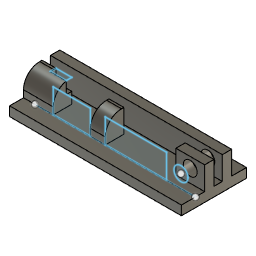
LM2596 Card Mount v10 (Autodesk Fusion 360 design; units mm, degrees)
Autodesk Fusion 360 part; units mm, degrees
note: some values were not read from the file. Chosen so that the rebuilt part matches the saved one: a direction; which face or edge a step refers to.
imported_body "Base Feature1'" makes body 1
sketch "Sketch1" plane through (0, 0, 0) normal (1, 0, 0) x (0, 1, 0)
  line L0 (7.8, 0) -> (0, 0)
  line L1 (0, 0) -> (0, 3.5)
  line L2 (3.5, 7) -> (7.8, 7)
  line L3 (7.8, 7) -> (7.8, 0)
  arc A0 (3.5, 7) -> (0, 3.5) centre (3.5, 3.5) ccw
  line L4 (4, 7) -> (4, 2)
  line L5 (4, 2) -> (5.8, 2)
  line L6 (5.8, 2) -> (5.8, 7)
  line L7 (4, 2) -> (0, 2) construction
  line L8 (4, 7) -> (2, 7)
  line L9 (2, 7) -> (2, 2)
  line L10 (2, 2) -> (4, 2)
  line L11 (4, 2) -> (4, 7)
  dimension "d9" = 7
  dimension "d11" = 3.5
  dimension "d12" = 4
  dimension "d13" = 1.8
  dimension "d27" = 2
  dimension "d37" = 2
  dimension "d50" = 2
  constraint horizontal L0
  constraint vertical L1
  constraint horizontal L2
  constraint vertical L3
  constraint tangent L1 A0
  constraint tangent L2 A0
  constraint coincident L2 L4.start
  constraint perpendicular L2 L4
  constraint perpendicular L4 L5
  constraint coincident L2 L6.end
  constraint perpendicular L2 L6
  constraint coincident L0.end L1.start
  constraint coincident L1 L7.end
  constraint collinear L5 L7
  constraint horizontal L8
  constraint vertical L9
  constraint horizontal L10
  constraint vertical L11
  measures "d9" distance of L0.start L2.end
  measures "d11" radius of A0
  measures "d12" distance of L1.end L4
  measures "d13" distance of L4 L6
  measures "d27" distance of L0 L5
  measures "d37" distance of L3 L6
  measures "d50" distance of L4.start L8.end
extrude "Extrude1" add sketch "Sketch1" along normal blind 37 separate body contours L0 L1 L2 L3 A0 L5 L6 L9 L10 | L2 A0 L4 L8 L9 L10 L11 sketch seen with x (1, 0, 0) y (0, 0, -1) z (0, 1, 0) at (0, -1.7661, 8.5008) makes body 2
sketch "Sketch2" plane through (0, 0, 0) normal (0, 1, 0) x (1, 0, 0)
  line L0 (6.4, -7.2451) -> (14.4, -7.2451)
  line L1 (14.4, -7.2451) -> (14.4, -2)
  line L2 (14.4, -2) -> (6.4, -2)
  line L3 (6.4, -2) -> (6.4, -7.2451)
  line L4 (17.6, -7.2451) -> (30.8, -7.2451)
  line L5 (30.8, -7.2451) -> (30.8, -2)
  line L6 (30.8, -2) -> (17.6, -2)
  line L7 (17.6, -2) -> (17.6, -7.2451)
  circle A0 centre (33.9, -4.8) radius 1.5
  line L8 (2.4997, -2) -> (37, -2)
  dimension "d16" = 3
  dimension "d17" = 2.8
  dimension "d24" = 2
  dimension "d34" = 13.2
  dimension "d35" = 3.2
  dimension "d36" = 8
  dimension "d53" = 6.2
  constraint perpendicular L3 L8
  constraint collinear L0 L4
  constraint collinear L2 L8
  constraint collinear L6 L8
  measures "d16" diameter of A0
  measures "d17" distance of L6 A0.centre
  measures "d24" distance of origin L8
  measures "d34" distance of L5 L7
  measures "d35" distance of L1 L7
  measures "d36" distance of L1 L3
  measures "d53" distance of L5 L8.end
extrude "Extrude2" cut sketch "Sketch2" along normal blind 4 contours L0 L1 L2 L3 L8 | L4 L5 L6 L7 L8 sketch seen with x (1, 0, 0) y (0, 0, -1) z (0, 1, 0) at (0, -1.7661, 8.5008) bodies 2
extrude "Extrude4" cut sketch "Sketch2" along normal blind 8 contours A0 sketch seen with x (1, 0, 0) y (0, 0, -1) z (0, 1, 0) at (0, -1.7661, 8.5008) bodies 2
sketch "Sketch3" plane through (0, 0, 0) normal (0, 0, 1) x (1, 0, 0)
  line L0 (0, 11) -> (37, 11)
  line L1 (37, 11) -> (37, -3)
  line L2 (37, -3) -> (0, -3)
  line L3 (0, -3) -> (0, 11)
  constraint horizontal L0
  constraint vertical L1
  constraint horizontal L2
  constraint vertical L3
sketch "Sketch4" plane through (0, 0, 0) normal (0, 0, 1) x (1, 0, 0)
  line L0 (6.4, 4, 7.0003) -> (3, 4, 7.0003)
  line L1 (3, 4, 7.0003) -> (3, 2.8, 7.0003)
  line L2 (3, 2.8, 7.0003) -> (6.4, 2.8, 7.0003)
  line L3 (6.4, 2.8, 7.0003) -> (6.4, 4, 7.0003)
  dimension "d46" = 3.4
  dimension "d47" = 1.2
sketch "Sketch4 (curves 7.0003 mm off its plane)" plane through (0, 0, 7.0003) normal (0, 0, 1) x (1, 0, 0)
  line L0 (6.4, 4) -> (3, 4)
  line L1 (3, 4) -> (3, 2.8)
  line L2 (3, 2.8) -> (6.4, 2.8)
  line L3 (6.4, 2.8) -> (6.4, 4)
extrude "Extrude7" cut sketch "Sketch4 (curves 7.0003 mm off its plane)" against normal blind 2.6 sketch seen with x (1, 0, 0) y (0, 0, -1) z (0, 1, 0) at (0, -1.7661, 8.5008) bodies 2
delete_face "DeleteFace1" 1 faces at (33.892, 4.8053, 6.6792) on bodies 2
ref_plane "WorkPlane1" through (0, 0, 2) normal (0, 0, 1) x (1, 0, 0)
split_face "SplitFace1" 1 faces at (2.1333, 0.0673, 8.5008) by plane through (0, 0.2339, 8.5008) normal (0, 1, 0) on bodies 2
move_face "OffsetFaces1" offset -2 1 faces at (31.3333, 2.8339, 8.5008) on bodies 2
extrude "Extrude8" add sketch "Sketch3" along normal blind 2 sketch seen with x (1, 0, 0) y (0, 0, -1) z (0, 1, 0) at (0, -1.7661, 8.5008) bodies 2
hidden bodies 1
